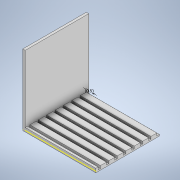
# Autodesk Inventor part: Part1
Saved by Autodesk Inventor 2022 (Build 260153000, 153)
## iProperties
Created: 2022-03-28
Part Number: Part1
Material: Generic
Document SubType Name: Modeling
Designer: Aditya Gupte
Density: 1 g/cm^3
Appearance: Default
Author: Aditya Gupte
Autodesk Inventor part; units mm, degrees
ref_plane "YZ Plane" through (0, 0, 0) normal (1, 0, 0) x (0, 1, 0)
ref_plane "XZ Plane" through (0, 0, 0) normal (0, 1, 0) x (-1, 0, 0)
ref_plane "XY Plane" through (0, 0, 0) normal (0, 0, 1) x (1, 0, 0)
sketch "Sketch1" plane through (0, 0, 0) normal (0, 0, 1) x (1, 0, 0)
  line L0 (0, 0) -> (15000, 0)
  line L1 (0, 0) -> (0, 14450)
  line L2 (0, 14450) -> (500, 14450)
  line L3 (500, 14450) -> (500, 300)
  line L4 (500, 300) -> (14950, 300)
  line L5 (14950, 300) -> (14950, 0)
  dimension "d0" = 15000
  dimension "d1" = 14450
  dimension "d2" = 500
  dimension "d3" = 14150
  dimension "d4" = 14450
  constraints: 12 end point, 3 perpendicular, 2 horizontal, 1 point on line, 1 vertical
  measures "d0" distance of L0.start L0.end
  measures "d1" distance of L0.start L1.end
  measures "d2" distance of L1.end L2.end
  measures "d3" distance of L2.end L3.end
  measures "d4" distance of L3.end L4.end
extrude "Extrusion1" add sketch "Sketch1" against normal blind 13000
sketch "Sketch2" plane through (500, 300, 0) normal (0, 1, 0) x (1, 0, 0)
  line L0 (14450, 0) -> (0, 0) projected
  line L1 (0, 0) -> (0, 13000) projected
  line L2 (-500, 0) -> (-500, 13000) projected
  dimension "d8" = 500
  measures "d8" distance between parallel lines of L1 L2
sketch "Sketch3" plane through (500, 300, 0) normal (0, 1, 0) x (1, 0, 0)
  line L0 (14450, 0) -> (14450, 13000) projected
  line L1 (14450, 0) -> (0, 0) projected
  line L2 (14450, 450) -> (0, 450)
  line L3 (14450, 950) -> (0, 950)
  line L4 (0, 0) -> (0, 13000) projected
  line L5 (0, 0) -> (0, 450)
  line L6 (14450, 0) -> (14450, 450)
  line L7 (0, 950) -> (14450, 950)
  line L8 (14450, 950) -> (14450, 2170)
  line L9 (14450, 2170) -> (0, 2170)
  line L10 (0, 2170) -> (0, 950)
  line L11 (0, 2670) -> (14450, 2670)
  line L12 (14450, 2670) -> (14450, 3890)
  line L13 (14450, 3890) -> (0, 3890)
  line L14 (0, 3890) -> (0, 2670)
  line L15 (0, 4390) -> (14450, 4390)
  line L16 (14450, 4390) -> (14450, 5610)
  line L17 (14450, 5610) -> (0, 5610)
  line L18 (0, 5610) -> (0, 4390)
  line L19 (0, 6110) -> (14450, 6110)
  line L20 (14450, 6110) -> (14450, 7330)
  line L21 (14450, 7330) -> (0, 7330)
  line L22 (0, 7330) -> (0, 6110)
  line L23 (0, 7830) -> (14450, 7830)
  line L24 (14450, 7830) -> (14450, 9050)
  line L25 (14450, 9050) -> (0, 9050)
  line L26 (0, 9050) -> (0, 7830)
  line L27 (0, 9550) -> (14450, 9550)
  line L28 (14450, 9550) -> (14450, 10770)
  line L29 (14450, 10770) -> (0, 10770)
  line L30 (0, 10770) -> (0, 9550)
  line L31 (0, 11270) -> (14450, 11270)
  line L32 (14450, 11270) -> (14450, 12490)
  line L33 (14450, 12490) -> (0, 12490)
  line L34 (0, 12490) -> (0, 11270)
  point P0 (-500, 0)
  point P1 (0, 5610)
  point P2 (0, 7330)
  point P3 (0, 10770)
  point P4 (0, 12490)
  dimension "d9" = 450
  dimension "d10" = 14450
  dimension "d11" = 14450
  dimension "d12" = 500
  dimension "d13" = 1220
  dimension "d14" = 500
  dimension "d15" = 1220
  dimension "d16" = 1220
  dimension "d17" = 500
  dimension "d18" = 1220
  dimension "d19" = 500
  dimension "d20" = 1220
  dimension "d21" = 500
  dimension "d22" = 1220
  dimension "d23" = 500
  dimension "d24" = 1220
  dimension "d25" = 500
  constraints: 64 end point, 14 parallel, 9 horizontal, 7 perpendicular, 1 vertical, 17 other
  measures "d9" distance from line of L2.start L1
  measures "d10" distance of L2.start L2.end
  measures "d11" distance of L3.start L3.end
  measures "d12" distance between parallel lines of L3 L2
  measures "d13" distance of L8.end L7.end
  measures "d14" distance between parallel lines of L11 L9
  measures "d15" distance of L11.end L12.end
  measures "d16" distance of L16.end L15.end
  measures "d17" distance between parallel lines of L15 L13
  measures "d18" distance of L20.end L19.end
  measures "d19" distance between parallel lines of L19 L17
  measures "d20" distance of L24.end L23.end
  measures "d21" distance between parallel lines of L23 L21
  measures "d22" distance of L28.end L27.end
  measures "d23" distance between parallel lines of L27 L25
  measures "d24" distance of L32.end L31.end
  measures "d25" distance between parallel lines of L31 L29
extrude "Extrusion2" add sketch "Sketch3" along normal blind 500 contours L3 L4 L9 L0 | L11 L4 L13 L0 | L15 L4 L17 L0 | L19 L4 L21 L0 | L23 L4 L25 L0 | L27 L4 L29 L0 | L31 L4 L33 L0
sketch "Sketch4" plane through (500, 300, 0) normal (0, 1, 0) x (1, 0, 0)
  line L0 (0, 0) -> (0, 13000) projected
  line L1 (14450, 0) -> (14450, 13000) projected
  line L2 (0, 0) -> (14450, 0)
  line L3 (14450, 0) -> (14450, 450)
  line L4 (14450, 450) -> (0, 450)
  line L5 (0, 450) -> (0, 0)
  point P0 (-500, 0)
  dimension "d28" = 450
  constraints: 8 end point, 2 parallel, 1 horizontal, 1 perpendicular, 1 point on line
  measures "d28" distance of L3.end L2.end
extrude "Extrusion3" add sketch "Sketch4" along normal blind 500
body "Solid1"
